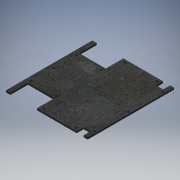
# Autodesk Inventor part: Blacha
Saved by Autodesk Inventor 2019 (Build 230136000, 136)
## iProperties
Created: 2021-12-21
Part Number: Blacha
Material: Stal
Document SubType Name: Modeling
Designer: Michał
Density: 7.85 g/cm^3
Appearance: Płyta
Mass: 120.709 g
Surface Area: 165.638 cm^2
Volume: 15.3769 cm^3
Author: Michał
Autodesk Inventor part; units mm, degrees
ref_plane "YZ Plane" through (0, 0, 0) normal (1, 0, 0) x (0, 1, 0)
ref_plane "XZ Plane" through (0, 0, 0) normal (0, 1, 0) x (-1, 0, 0)
ref_plane "XY Plane" through (0, 0, 0) normal (0, 0, 1) x (1, 0, 0)
sketch "Szkic1" plane through (0, 0, 0) normal (0, 1, 0) x (-1, 0, 0)
  line L0 (0, 0) -> (92.7, 0)
  line L1 (92.7, 0) -> (92.7, -98)
  line L2 (92.7, -98) -> (0, -98)
  line L3 (0, -98) -> (0, 0)
  line L4 (4.5, -98) -> (12.5, -98)
  line L5 (12.5, -98) -> (12.5, -90.1)
  line L6 (12.5, -90.1) -> (4.5, -90.1)
  line L7 (4.5, -90.1) -> (4.5, -98)
  line L8 (57.5, -98) -> (87.7, -98)
  line L9 (87.7, -98) -> (87.7, -78)
  line L10 (87.7, -78) -> (57.5, -78)
  line L11 (57.5, -78) -> (57.5, -98)
  line L12 (92.7, -49) -> (0, -49) construction
  line L13 (92.7, 0) -> (0, 0)
  line L14 (4.5, 0) -> (12.5, 0)
  line L15 (12.5, 0) -> (12.5, -7.9)
  line L16 (12.5, -7.9) -> (4.5, -7.9)
  line L17 (4.5, -7.9) -> (4.5, 0)
  line L18 (57.5, 0) -> (87.7, 0)
  line L19 (87.7, 0) -> (87.7, -20)
  line L20 (87.7, -20) -> (57.5, -20)
  line L21 (57.5, -20) -> (57.5, 0)
  dimension "d0" = 92.7
  dimension "d1" = 98
  dimension "d2" = 57.5
  dimension "d3" = 30.2
  dimension "d4" = 20
  dimension "d5" = 7.9
  dimension "d6" = 8
  dimension "d8" = 4.5
  constraints: 44 end point, 8 symmetric about line, 6 parallel, 4 point on line, 3 horizontal, 3 perpendicular, 2 midpoint
  measures "d0" distance between parallel lines of L3 L1
  measures "d1" distance between parallel lines of L0 L2
  measures "d2" distance between parallel lines of L3 L11
  measures "d3" distance between parallel lines of L11 L9
  measures "d4" distance between parallel lines of L2 L10
  measures "d5" distance between parallel lines of L2 L6
  measures "d6" distance between parallel lines of L5 L7
  measures "d8" distance between parallel lines of L3 L7
extrude "Wyciągnięcie proste1" add sketch "Szkic1" along normal blind 2 contours L0 L17 L16 L15 L21 L20 L19 L1 L2 L9 L10 L11 L5 L6 L7 L3
sketch "Szkic2" plane through (0, 2, 0) normal (0, 1, 0) x (1, 0, 0)
  line L0 (0, 0) -> (0, 98) construction
  line L1 (0, 49) -> (-92.7, 49) construction
  line L2 (-92.7, 98) -> (-92.7, 0) construction
  line L3 (-2.2, 49) -> (-2.2, 87.6) construction
  line L4 (-52.4, 94.75) -> (-15.8, 94.75) construction
  line L5 (-87.45, 74.6) -> (-58.85, 74.6) construction
  line L6 (-87.45, 49) -> (-87.45, 74.6) construction
  line L7 (-57.5, 78) -> (-87.7, 78) construction
  line L8 (-12.5, 98) -> (-57.5, 98) construction
  line L9 (-12.5, 90.1) -> (-12.5, 98) construction
  line L10 (-52.4, 3.25) -> (-15.8, 3.25) construction
  line L11 (-87.45, 23.4) -> (-58.85, 23.4) construction
  line L12 (-57.5, 20) -> (-87.7, 20) construction
  line L13 (-12.5, 0) -> (-57.5, 0) construction
  line L14 (-12.5, 7.9) -> (-12.5, 0) construction
  point P0 (-2.2, 10.4)
  point P1 (-50.7, 74.6)
  dimension "d11" = 2.2
  dimension "d12" = 38.6
  dimension "d13" = 3.25
  dimension "d14" = 3.3
  dimension "d15" = 36.6
  dimension "d16" = 3.4
  dimension "d17" = 5.25
  dimension "d18" = 28.6
  dimension "d26" = 42
  constraints: 20 end point, 10 symmetric about line, 3 point on line, 2 horizontal, 2 midpoint, 2 parallel, 2 vertical
  measures "d11" distance from line of L0 L3.end
  measures "d12" distance of L3.start L3.end
  measures "d13" distance between parallel lines of L8 L4
  measures "d14" distance from line of L9 L4.end
  measures "d15" distance of L4.start L4.end
  measures "d16" distance between parallel lines of L7 L5
  measures "d17" distance from line of L2 L5.start
  measures "d18" distance of L5.start L5.end
  measures "d26" distance from line of L2 point (-50.7, 74.6)
hole "Otwór1" at (-2.2, 2, -87.6) at (-2.2, 2, -49) at (-15.8, 2, -94.75) at (-52.4, 2, -94.75) at (-58.85, 2, -74.6) at (-87.45, 2, -74.6) at (-87.45, 2, -49) at (-52.4, 2, -3.25) at (-15.8, 2, -3.25) at (-87.45, 2, -23.4) at (-58.85, 2, -23.4) at (-2.2, 2, -10.4) at (-50.7, 2, -74.6) direction (0, -1, 0) diameter 2.459 end through all thread size "M3x0.5" class "6H" standard "ISO Metric profile"
